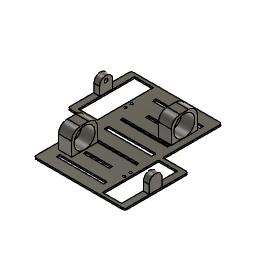
Chassis V4.1 (Autodesk Fusion 360 design; units mm, degrees)
Autodesk Fusion 360 part; units mm, degrees
note: some values were not read from the file. Chosen so that the rebuilt part matches the saved one: which face or edge a step refers to. Set by a fixed rule: which sketch regions a step uses.
sketch "Sketch1" plane through (0, 0, 0) normal (0, 0, 1) x (1, 0, 0)
  line L0 (0, 0) -> (135, 0)
  line L1 (135, 0) -> (135, 150)
  line L2 (135, 150) -> (0, 150)
  line L3 (0, 150) -> (0, 0)
  dimension "d1" = 135
  dimension "d2" = 150
  constraint horizontal L0
  constraint vertical L1
  constraint horizontal L2
  constraint vertical L3
  constraint coincident L0.start L3.end
  measures "d1" distance of L0.start L0.end
  measures "d2" distance of L0.start L2.end
extrude "Extrude1" add sketch "Sketch1" along normal blind 1.75 makes body 1
sketch "Sketch2" plane through (0, 0, 1.75) normal (0, 0, 1) x (-1, 0, 0)
  line L0 (0, -150) -> (0, 0)
  line L1 (0, 0) -> (-135, 0)
  line L2 (-135, 0) -> (-135, -150)
  line L3 (-135, -150) -> (0, -150)
  line L4 (-7.5, -7.5) -> (-127.5, -7.5)
  line L5 (-127.5, -7.5) -> (-127.5, -142.5)
  line L6 (-127.5, -142.5) -> (-7.5, -142.5)
  line L7 (-7.5, -142.5) -> (-7.5, -7.5)
  line L8 (-7.5, -142.5) -> (-29.5, -142.5)
  line L9 (-29.5, -142.5) -> (-29.5, -77.5)
  line L10 (-29.5, -77.5) -> (-7.5, -77.5)
  line L11 (-7.5, -77.5) -> (-7.5, -142.5)
  line L12 (-127.5, -142.5) -> (-127.5, -77.5)
  line L13 (-105.5, -142.5) -> (-127.5, -142.5)
  line L14 (-127.5, -77.5) -> (-105.5, -77.5)
  line L15 (-105.5, -77.5) -> (-105.5, -142.5)
  line L16 (-29.5, -72.5) -> (-29.5, -7.5)
  line L17 (-7.5, -72.5) -> (-29.5, -72.5)
  line L18 (-29.5, -7.5) -> (-7.5, -7.5)
  line L19 (-7.5, -7.5) -> (-7.5, -72.5)
  line L20 (-127.5, -72.5) -> (-127.5, -7.5)
  line L21 (-105.5, -72.5) -> (-127.5, -72.5)
  line L22 (-127.5, -7.5) -> (-105.5, -7.5)
  line L23 (-105.5, -7.5) -> (-105.5, -72.5)
  dimension "d5" = -7.5
  dimension "d6" = 22
  dimension "d7" = 65
  dimension "d10" = -98
  dimension "d11" = 70
  constraint horizontal L8
  constraint vertical L9
  constraint horizontal L10
  constraint vertical L11
  measures "d6" distance of L6.end L8.end
  measures "d7" distance of L6.end L10.end
extrude "Extrude2" cut sketch "Sketch2" against normal up to surface (1.75 mm away) contours L4 L7 L16 L17 L18 L19 | L4 L5 L20 L21 L22 L23 | L6 L7 L8 L9 L10 L11 | L5 L6 L12 L13 L14 L15 bodies 1
sketch "Sketch3" plane through (0, 0, 1.75) normal (0, 0, 1) x (-1, 0, 0)
  line L0 (-127.5, -72.5) -> (-127.5, -7.5)
  line L1 (-127.5, -7.5) -> (-105.5, -7.5)
  line L2 (-105.5, -142.5) -> (-127.5, -142.5)
  line L3 (-127.5, -142.5) -> (-127.5, -77.5)
  line L4 (-127.5, -77.5) -> (-105.5, -77.5)
  line L5 (-7.5, -77.5) -> (-7.5, -142.5)
  line L6 (-7.5, -142.5) -> (-29.5, -142.5)
  line L7 (-29.5, -142.5) -> (-29.5, -77.5)
  line L8 (-29.5, -77.5) -> (-7.5, -77.5)
  line L9 (-7.5, -7.5) -> (-7.5, -72.5)
  line L10 (-29.5, -72.5) -> (-29.5, -7.5)
  line L11 (-29.5, -7.5) -> (-7.5, -7.5)
  line L12 (0, -150) -> (0, 0)
  line L13 (0, 0) -> (-135, 0)
  line L14 (-135, 0) -> (-135, -150)
  line L15 (-135, -150) -> (0, -150)
  line L16 (-29.5, -110) -> (-110.5, -110) construction
  line L17 (-29.5, -40) -> (-110.5, -40) construction
  line L18 (-29.5, -110) -> (-33.25, -110) construction
  line L19 (-30.0705, -117.5) -> (-36.4295, -117.5)
  line L20 (-36.4295, -117.5) -> (-36.4295, -102.5)
  line L21 (-36.4295, -102.5) -> (-30.0705, -102.5)
  line L22 (-30.0705, -102.5) -> (-30.0705, -117.5)
  line L23 (-30.0705, -117.5) -> (-36.4295, -102.5) construction
  line L24 (-36.4295, -117.5) -> (-30.0705, -102.5) construction
  line L25 (-98.5705, -47.5) -> (-104.9295, -47.5)
  line L26 (-98.5705, -32.5) -> (-98.5705, -47.5)
  line L27 (-104.9295, -32.5) -> (-98.5705, -32.5)
  line L28 (-104.9295, -47.5) -> (-104.9295, -32.5)
  line L29 (-110.5, -110) -> (-135, -110) construction
  line L30 (-33.25, -117.5) -> (-33.25, -110) construction
  line L31 (-33.25, -110) -> (-33.25, -102.5) construction
  circle A0 centre (-33.25, -113.75) radius 1.5
  circle A1 centre (-33.25, -106.25) radius 1.5
  line L32 (-101.75, -47.5) -> (-101.75, -40) construction
  line L33 (-101.75, -40) -> (-101.75, -32.5) construction
  circle A2 centre (-101.75, -43.75) radius 1.5
  circle A3 centre (-101.75, -36.25) radius 1.5
  line L34 (-7.5, -110) -> (0, -110) construction
  line L35 (-7.0568, -117.5) -> (-0.4432, -117.5)
  line L36 (-0.4432, -117.5) -> (-0.4432, -102.5)
  line L37 (-0.4432, -102.5) -> (-7.0568, -102.5)
  line L38 (-7.0568, -102.5) -> (-7.0568, -117.5)
  line L39 (-7.0568, -117.5) -> (-0.4432, -102.5) construction
  line L40 (-0.4432, -117.5) -> (-7.0568, -102.5) construction
  line L41 (-134.5568, -47.5) -> (-127.9432, -47.5)
  line L42 (-134.5568, -32.5) -> (-134.5568, -47.5)
  line L43 (-127.9432, -32.5) -> (-134.5568, -32.5)
  line L44 (-127.9432, -47.5) -> (-127.9432, -32.5)
  line L45 (-105.5, -72.5) -> (-127.5, -72.5)
  line L46 (-7.5, -72.5) -> (-29.5, -72.5)
  line L47 (-105.5, -77.5) -> (-105.5, -142.5)
  line L48 (-105.5, -7.5) -> (-105.5, -72.5)
  point P0 (-33.25, -110)
  point P1 (-3.75, -110)
  dimension "d14" = 3.75
  dimension "d15" = 15
  dimension "d18" = -68.5
  dimension "d19" = 70
  dimension "d26" = 3
  dimension "d27" = 3
  dimension "d28" = 3
  dimension "d29" = 3
  dimension "d49" = 15
  dimension "d52" = -127.5
  dimension "d53" = 70
  constraint midpoint L7 L16.start
  constraint midpoint L10 L17.start
  constraint perpendicular L7 L18
  constraint horizontal L19
  constraint perpendicular L19 L20
  constraint parallel L19 L21
  constraint parallel L20 L22
  constraint coincident L23 P0
  constraint coincident L24 P0
  constraint coincident P0 L18.end
  constraint coincident L14 L29.end
  constraint perpendicular L14 L29
  constraint midpoint L19 L30.start
  constraint midpoint L21 L31.end
  constraint midpoint L30 A0.centre
  constraint midpoint L31 A1.centre
  constraint midpoint L25 L32.start
  constraint coincident L17 L32.end
  constraint perpendicular L17 L32
  constraint midpoint L27 L33.end
  constraint midpoint L32 A2.centre
  constraint midpoint L33 A3.centre
  constraint midpoint L5 L34.start
  constraint coincident L12 L34.end
  constraint perpendicular L12 L34
  constraint horizontal L35
  constraint perpendicular L35 L36
  constraint parallel L35 L37
  constraint parallel L36 L38
  constraint coincident L39 P1
  constraint coincident L40 P1
  constraint midpoint L34 P1
  measures "d14" distance of L16.start P0
  measures "d15" distance of L19.end L20.end
  measures "d26" diameter of A0
  measures "d27" diameter of A1
  measures "d28" diameter of A2
  measures "d29" diameter of A3
  measures "d49" distance of L35.end L36.end
extrude "Extrude3" add sketch "Sketch3" along normal blind 17.5 contours L35 L36 L37 L38 | L41 L42 L43 L44 bodies 1
extrude "Extrude4" cut sketch "Sketch3" against normal up to surface (1.75 mm away) contours A0 | A1 | A2 | A3 bodies 1
sketch "Sketch4" plane through (127.5, 0, 0) normal (-1, 0, 0) x (0, -1, 0)
  line L0 (-72.5, 0) -> (-7.5, 0)
  line L1 (-7.5, 0) -> (-7.5, 1.75)
  line L2 (-72.5, 1.75) -> (-7.5, 1.75) construction
  line L3 (-40, 1.75) -> (-40, 13.875) construction
  circle A0 centre (-40, 13.875) radius 2.15
  line L4 (-72.5, 1.75) -> (-72.5, 0)
  line L5 (-7.5, 1.75) -> (-72.5, 1.75)
  dimension "d32" = 12.125
  dimension "d33" = 4.3
  constraint midpoint L2 L3.start
  constraint coincident L3.end A0.centre
  measures "d32" distance of L3.start L3.end
  measures "d33" diameter of A0
sketch "Sketch5" plane through (7.5, 0, 0) normal (1, 0, 0) x (0, 1, 0)
  line L0 (77.5, 0) -> (142.5, 0)
  line L1 (142.5, 0) -> (142.5, 1.75)
  line L2 (77.5, 1.75) -> (77.5, 0)
  line L3 (110, 1.75) -> (110, 13.875) construction
  circle A0 centre (110, 13.875) radius 2.15
  line L4 (142.5, 1.75) -> (77.5, 1.75)
  dimension "d34" = 12.125
  dimension "d35" = 4.3
  constraint coincident L3.end A0.centre
  constraint midpoint L3.start L4
  constraint perpendicular L3 L4
  measures "d34" distance of L3.start L3.end
  measures "d35" diameter of A0
extrude "Extrude5" cut sketch "Sketch5" against normal blind 5 contours A0 bodies 1
extrude "Extrude6" cut sketch "Sketch4" against normal blind 5 contours A0 bodies 1
sketch "Sketch6" plane through (0, 0, 1.75) normal (0, 0, 1) x (-1, 0, 0)
  line L0 (-107.9876, -110) -> (-100.4877, -110.0388) construction
  line L1 (-100.4877, -110.0388) -> (-80.4879, -109.9612) construction
  line L2 (-97.9878, -125) -> (-82.9878, -125)
  line L3 (-82.9878, -125) -> (-82.9878, -95)
  line L4 (-82.9878, -95) -> (-97.9878, -95)
  line L5 (-97.9878, -95) -> (-97.9878, -125)
  line L6 (-97.9878, -125) -> (-82.9878, -95) construction
  line L7 (-82.9878, -125) -> (-97.9878, -95) construction
  line L8 (0, 0) -> (-135, 0)
  line L9 (-69.9889, -150) -> (-67.5, 0) construction
  line L10 (0, -150) -> (0, 0)
  line L11 (-135, 0) -> (-135, -150)
  line L12 (0, -75) -> (-135, -75) construction
  line L13 (-51.9878, -55) -> (-36.9878, -55)
  line L14 (-51.9878, -25) -> (-51.9878, -55)
  line L15 (-36.9878, -25) -> (-51.9878, -25)
  line L16 (-36.9878, -55) -> (-36.9878, -25)
  line L17 (-29.5, -110) -> (-37, -110) construction
  line L18 (-37, -110) -> (-107.9876, -110) construction
  point P0 (-90.4878, -110)
  dimension "d40" = 7.5
  dimension "d41" = 20
  dimension "d42" = 15
  dimension "d43" = 30
  dimension "d46" = 46
  dimension "d47" = 70
  dimension "d48" = 7.5
  constraint horizontal L2
  constraint perpendicular L2 L3
  constraint parallel L2 L4
  constraint parallel L3 L5
  constraint coincident L6 P0
  constraint coincident L7 P0
  constraint midpoint L1 P0
  constraint midpoint L8 L9.end
  constraint midpoint L10 L12.start
  constraint midpoint L11 L12.end
  constraint perpendicular L5 L18
  measures "d40" distance of L0.end L0.start
  measures "d41" distance of L0.end L1.end
  measures "d42" distance of L3.end L4.end
  measures "d43" distance of L2.end L3.end
  measures "d48" distance of L17.start L17.end
extrude "Extrude7" add sketch "Sketch6" along normal blind 26 bodies 1
sketch "Sketch7" plane through (51.9878, 0, 0) normal (1, 0, 0) x (0, 1, 0)
  line L0 (25, 1.75) -> (55, 1.75)
  line L1 (55, 1.75) -> (55, 27.75)
  line L2 (55, 27.75) -> (25, 27.75)
  line L3 (25, 27.75) -> (25, 1.75)
  line L4 (40, 1.75) -> (40, 26) construction
  circle A0 centre (40, 13.875) radius 12.125
  dimension "d56" = 24.25
  dimension "d57" = 24.25
  constraint midpoint L0 L4.start
  constraint perpendicular L0 L4
  constraint midpoint L4 A0.centre
  measures "d56" distance of L4.start L4.end
  measures "d57" diameter of A0
sketch "Sketch8" plane through (82.9878, 0, 0) normal (-1, 0, 0) x (0, -1, 0)
  line L0 (-125, 1.75) -> (-95, 1.75)
  line L1 (-95, 1.75) -> (-95, 27.75)
  line L2 (-95, 27.75) -> (-125, 27.75)
  line L3 (-125, 27.75) -> (-125, 1.75)
  line L4 (-110, 1.75) -> (-110, 26) construction
  circle A0 centre (-110, 13.875) radius 12.125
  dimension "d58" = 24.25
  dimension "d59" = 24.25
  constraint midpoint L0 L4.start
  constraint perpendicular L0 L4
  constraint midpoint L4 A0.centre
  measures "d58" distance of L4.start L4.end
  measures "d59" diameter of A0
extrude "Extrude8" cut sketch "Sketch8" against normal up to surface (15 mm away) contours A0 bodies 1
extrude "Extrude9" cut sketch "Sketch7" against normal blind 15 contours A0 bodies 1
fillet "Fillet1" [suppressed]
fillet "Fillet4" radius 10 4 edges at (90.4878, 95, 27.75) (90.4878, 125, 27.75) (44.4878, 55, 27.75) (44.4878, 25, 27.75) on bodies 1
fillet "Fillet5" radius 7.5 4 edges at (131.25, 47.5, 19.25) (131.25, 32.5, 19.25) (3.75, 102.5, 19.25) (3.75, 117.5, 19.25) on bodies 1
sketch "Sketch9" plane through (0, 0, 0) normal (0, 0, -1) x (1, 0, 0)
  circle A0 centre (33.25, -106.25) radius 1.5
  circle A1 centre (33.25, -113.75) radius 1.5
  line L0 (105.5, -77.5) -> (127.5, -77.5)
  line L1 (127.5, -77.5) -> (127.5, -142.5)
  line L2 (127.5, -142.5) -> (105.5, -142.5)
  line L3 (7.5, -72.5) -> (7.5, -7.5)
  line L4 (7.5, -7.5) -> (29.5, -7.5)
  line L5 (29.5, -7.5) -> (29.5, -72.5)
  line L6 (29.5, -72.5) -> (7.5, -72.5)
  line L7 (105.5, -7.5) -> (127.5, -7.5)
  line L8 (127.5, -7.5) -> (127.5, -72.5)
  line L9 (127.5, -72.5) -> (105.5, -72.5)
  line L10 (7.5, -142.5) -> (7.5, -77.5)
  line L11 (7.5, -77.5) -> (29.5, -77.5)
  line L12 (29.5, -77.5) -> (29.5, -142.5)
  line L13 (29.5, -142.5) -> (7.5, -142.5)
  line L14 (70, 0) -> (70, -150) construction
  line L15 (0, -75) -> (140, -75) construction
  line L16 (0, 0) -> (0, -75) construction
  line L17 (0, 0) -> (0, -75) construction
  line L18 (0, -37.5) -> (140, -37.5) construction
  line L19 (0, -75) -> (0, -145) construction
  line L20 (0, -110) -> (140, -110) construction
  line L21 (85, -35.75) -> (55, -35.75)
  line L22 (55, -35.75) -> (55, -39.25)
  line L23 (55, -39.25) -> (85, -39.25)
  line L24 (85, -39.25) -> (85, -35.75)
  line L25 (85, -35.75) -> (55, -39.25) construction
  line L26 (55, -35.75) -> (85, -39.25) construction
  line L27 (97.5, -72.5) -> (42.5, -72.5)
  line L28 (42.5, -72.5) -> (42.5, -77.5)
  line L29 (42.5, -77.5) -> (97.5, -77.5)
  line L30 (97.5, -77.5) -> (97.5, -72.5)
  line L31 (97.5, -72.5) -> (42.5, -77.5) construction
  line L32 (42.5, -72.5) -> (97.5, -77.5) construction
  line L33 (85, -108.25) -> (55, -108.25)
  line L34 (55, -108.25) -> (55, -111.75)
  line L35 (55, -111.75) -> (85, -111.75)
  line L36 (85, -111.75) -> (85, -108.25)
  line L37 (85, -108.25) -> (55, -111.75) construction
  line L38 (55, -108.25) -> (85, -111.75) construction
  line L39 (0, 0) -> (0, -37.5) construction
  line L40 (0, -37.5) -> (0, -75) construction
  line L41 (0, -75) -> (0, -110) construction
  line L42 (0, -110) -> (0, -151) construction
  line L43 (0, -18.75) -> (140, -18.75) construction
  line L44 (0, -56.25) -> (140, -56.25) construction
  line L45 (0, -92.5) -> (140, -92.5) construction
  line L46 (0, -130.5) -> (140, -130.5) construction
  line L47 (97.5, -54.875) -> (42.5, -54.875)
  line L48 (42.5, -54.875) -> (42.5, -57.625)
  line L49 (42.5, -57.625) -> (97.5, -57.625)
  line L50 (97.5, -57.625) -> (97.5, -54.875)
  line L51 (97.5, -54.875) -> (42.5, -57.625) construction
  line L52 (42.5, -54.875) -> (97.5, -57.625) construction
  line L53 (97.5, -91) -> (42.5, -91)
  line L54 (42.5, -91) -> (42.5, -94)
  line L55 (42.5, -94) -> (97.5, -94)
  line L56 (97.5, -94) -> (97.5, -91)
  line L57 (97.5, -91) -> (42.5, -94) construction
  line L58 (42.5, -91) -> (97.5, -94) construction
  line L59 (97.5, -128.5) -> (42.5, -128.5)
  line L60 (42.5, -128.5) -> (42.5, -132.5)
  line L61 (42.5, -132.5) -> (97.5, -132.5)
  line L62 (97.5, -132.5) -> (97.5, -128.5)
  line L63 (97.5, -128.5) -> (42.5, -132.5) construction
  line L64 (42.5, -128.5) -> (97.5, -132.5) construction
  line L65 (97.5, -16.75) -> (42.5, -16.75)
  line L66 (42.5, -16.75) -> (42.5, -20.75)
  line L67 (42.5, -20.75) -> (97.5, -20.75)
  line L68 (97.5, -20.75) -> (97.5, -16.75)
  line L69 (97.5, -16.75) -> (42.5, -20.75) construction
  line L70 (42.5, -16.75) -> (97.5, -20.75) construction
  line L71 (7.5, -72.5) -> (0, -72.5)
  line L72 (0, -72.5) -> (0, -7.3593)
  line L73 (0, -7.3593) -> (7.5, -7.3593)
  line L74 (7.5, -7.3593) -> (7.5, -72.5)
  line L75 (127.5, -77.5) -> (140, -77.5)
  line L76 (140, -77.5) -> (140, -142.564)
  line L77 (140, -142.564) -> (127.5, -142.564)
  line L78 (127.5, -142.564) -> (127.5, -77.5)
  line L79 (29.5, -7.5) -> (0, -7.5)
  line L80 (0, -7.5) -> (0, 0)
  line L81 (0, 0) -> (29.5, 0)
  line L82 (29.5, 0) -> (29.5, -7.5)
  line L83 (105.5, -142.5) -> (140, -142.5)
  line L84 (140, -142.5) -> (140, -150.5046)
  line L85 (140, -150.5046) -> (105.5, -150.5046)
  line L86 (105.5, -150.5046) -> (105.5, -142.5)
  line L87 (0, -150) -> (135, -150)
  line L88 (135, -150) -> (135, 0)
  line L89 (135, 0) -> (0, 0)
  line L90 (0, 0) -> (0, -150)
  line L91 (105.5, -72.5) -> (105.5, -7.5)
  line L92 (105.5, -142.5) -> (105.5, -77.5)
  circle A2 centre (101.75, -43.75) radius 1.5
  circle A3 centre (101.75, -36.25) radius 1.5
  point P0 (70, -37.5)
  point P1 (70, -75)
  point P2 (70, -110)
  point P3 (70, -56.25)
  point P4 (70, -92.5)
  point P5 (70, -130.5)
  point P6 (70, -18.75)
  dimension "d74" = 30
  dimension "d75" = 3.5
  dimension "d76" = 55
  dimension "d77" = 5
  dimension "d78" = 30
  dimension "d79" = 3.5
  dimension "d82" = 55
  dimension "d83" = 2.75
  dimension "d84" = 55
  dimension "d85" = 3
  dimension "d86" = 55
  dimension "d87" = 4
  dimension "d88" = 55
  dimension "d89" = 4
  constraint coincident L16.start L17.start
  constraint midpoint L17 L18.start
  constraint midpoint L19 L20.start
  constraint horizontal L21
  constraint perpendicular L21 L22
  constraint parallel L21 L23
  constraint parallel L22 L24
  constraint coincident L25 P0
  constraint coincident L26 P0
  constraint midpoint L18 P0
  constraint horizontal L27
  constraint perpendicular L27 L28
  constraint parallel L27 L29
  constraint parallel L28 L30
  constraint coincident L31 P1
  constraint coincident L32 P1
  constraint midpoint L14 P1
  constraint horizontal L33
  constraint perpendicular L33 L34
  constraint parallel L33 L35
  constraint parallel L34 L36
  constraint coincident L37 P2
  constraint coincident L38 P2
  constraint midpoint L20 P2
  constraint midpoint L39 L43.start
  constraint midpoint L40 L44.start
  constraint midpoint L41 L45.start
  constraint midpoint L42 L46.start
  constraint horizontal L47
  constraint perpendicular L47 L48
  constraint parallel L47 L49
  constraint parallel L48 L50
  constraint coincident L51 P3
  constraint coincident L52 P3
  constraint midpoint L44 P3
  constraint horizontal L53
  constraint perpendicular L53 L54
  constraint parallel L53 L55
  constraint parallel L54 L56
  constraint coincident L57 P4
  constraint coincident L58 P4
  constraint midpoint L45 P4
  constraint horizontal L59
  constraint perpendicular L59 L60
  constraint parallel L59 L61
  constraint parallel L60 L62
  constraint coincident L63 P5
  constraint coincident L64 P5
  constraint midpoint L46 P5
  constraint horizontal L65
  constraint perpendicular L65 L66
  constraint parallel L65 L67
  constraint parallel L66 L68
  constraint coincident L69 P6
  constraint coincident L70 P6
  constraint midpoint L43 P6
  constraint horizontal L71
  constraint vertical L72
  constraint horizontal L73
  constraint vertical L74
  constraint coincident L39 L72.end
  constraint coincident L3.start L6.end
  constraint horizontal L75
  constraint vertical L76
  constraint horizontal L77
  constraint vertical L78
  constraint coincident L0.end L1.start
  constraint horizontal L79
  constraint vertical L80
  constraint horizontal L81
  constraint vertical L82
  constraint coincident L4.end L5.start
  constraint horizontal L83
  constraint vertical L84
  constraint horizontal L85
  constraint vertical L86
  constraint coincident L2.end L83.start
  measures "d74" distance of L22.end L23.end
  measures "d75" distance of L21.end L22.end
  measures "d76" distance of L28.end L29.end
  measures "d77" distance of L27.end L28.end
  measures "d78" distance of L34.end L35.end
  measures "d79" distance of L33.end L34.end
  measures "d82" distance of L48.end L49.end
  measures "d83" distance of L47.end L48.end
  measures "d84" distance of L54.end L55.end
  measures "d85" distance of L53.end L54.end
  measures "d86" distance of L60.end L61.end
  measures "d87" distance of L59.end L60.end
  measures "d88" distance of L66.end L67.end
  measures "d89" distance of L65.end L66.end
extrude "Extrude10" cut sketch "Sketch9" against normal up to surface (1.75 mm away) contours L21 L22 L23 L24 | L27 L28 L29 L30 | L33 L34 L35 L36 | L47 L48 L49 L50 | L53 L54 L55 L56 | L59 L60 L61 L62 | L65 L66 L67 L68 bodies 1
extrude "Extrude11" cut sketch "Sketch9" against normal up to surface (1.75 mm away) contours L1 L75 L78 L83 L88 | L2 L77 L78 L83 L86 L87 L88 | L77 L78 L83 L88 | L77 L84 L85 L86 L87 L88 | L4 L73 L74 L79 L80 L81 L82 L89 L90 | L3 L71 L72 L74 L79 L90 | L72 L73 L74 L79 L80 L90 bodies 1
fillet "Fillet6" [suppressed]
sketch "Sketch10" plane through (0, 0, 0) normal (0, 0, -1) x (1, 0, 0)
  line L0 (0, -72.5) -> (0, -150)
  line L1 (0, -150) -> (105.5, -150)
  line L2 (105.5, -150) -> (105.5, -77.5)
  line L3 (105.5, -77.5) -> (135, -77.5)
  line L4 (135, -77.5) -> (135, 0)
  line L5 (135, 0) -> (29.5, 0)
  line L6 (29.5, 0) -> (29.5, -72.5)
  line L7 (29.5, -72.5) -> (0, -72.5)
  line L8 (7.5, -142.5) -> (7.5, -77.5)
  line L9 (7.5, -77.5) -> (29.5, -77.5)
  line L10 (29.5, -77.5) -> (29.5, -142.5)
  line L11 (29.5, -142.5) -> (7.5, -142.5)
  line L12 (105.5, -7.5) -> (127.5, -7.5)
  line L13 (127.5, -7.5) -> (127.5, -72.5)
  line L14 (127.5, -72.5) -> (105.5, -72.5)
  circle A0 centre (33.25, -113.75) radius 1.5
  circle A1 centre (33.25, -106.25) radius 1.5
  line L15 (97.5, -132.5) -> (42.5, -132.5)
  line L16 (42.5, -132.5) -> (42.5, -128.5)
  line L17 (42.5, -128.5) -> (97.5, -128.5)
  line L18 (97.5, -128.5) -> (97.5, -132.5)
  line L19 (85, -111.75) -> (55, -111.75)
  line L20 (55, -111.75) -> (55, -108.25)
  line L21 (55, -108.25) -> (85, -108.25)
  line L22 (85, -108.25) -> (85, -111.75)
  line L23 (97.5, -77.5) -> (42.5, -77.5)
  line L24 (42.5, -77.5) -> (42.5, -72.5)
  line L25 (42.5, -72.5) -> (97.5, -72.5)
  line L26 (97.5, -72.5) -> (97.5, -77.5)
  line L27 (97.5, -94) -> (42.5, -94)
  line L28 (42.5, -94) -> (42.5, -91)
  line L29 (42.5, -91) -> (97.5, -91)
  line L30 (97.5, -91) -> (97.5, -94)
  line L31 (97.5, -20.75) -> (42.5, -20.75)
  line L32 (42.5, -20.75) -> (42.5, -16.75)
  line L33 (42.5, -16.75) -> (97.5, -16.75)
  line L34 (97.5, -16.75) -> (97.5, -20.75)
  line L35 (85, -39.25) -> (55, -39.25)
  line L36 (55, -39.25) -> (55, -35.75)
  line L37 (55, -35.75) -> (85, -35.75)
  line L38 (85, -35.75) -> (85, -39.25)
  line L39 (97.5, -57.625) -> (42.5, -57.625)
  line L40 (42.5, -57.625) -> (42.5, -54.875)
  line L41 (42.5, -54.875) -> (97.5, -54.875)
  line L42 (97.5, -54.875) -> (97.5, -57.625)
  line L43 (105.5, -7.5) -> (105.5, 0) construction
  line L44 (29.5, -142.5) -> (29.5, -150) construction
  line L45 (29.5, -150) -> (31.5, -150) construction
  line L46 (31.5, -150) -> (36.5, -150)
  line L47 (36.5, -150) -> (36.5, 0)
  line L48 (36.5, 0) -> (31.5, 0)
  line L49 (31.5, 0) -> (31.5, -150)
  line L50 (105.5, 0) -> (103.5, 0) construction
  line L51 (103.5, 0) -> (98.5, 0)
  line L52 (98.5, 0) -> (98.5, -150)
  line L53 (98.5, -150) -> (103.5, -150)
  line L54 (103.5, -150) -> (103.5, 0)
  circle A2 centre (33.25, -113.75) radius 1.75
  circle A3 centre (33.25, -106.25) radius 1.75
  circle A4 centre (106.75, -36.25) radius 1.75
  circle A5 centre (101.75, -43.75) radius 1.75
  line L55 (33.25, -113.75) -> (33.25, -116.75)
  line L56 (33.25, -106.25) -> (33.25, -103.25)
  line L57 (36.5, -103.25) -> (31.5, -103.25)
  line L58 (36.5, -116.75) -> (31.5, -116.75)
  line L59 (106.75, -36.25) -> (106.75, -33.25)
  line L60 (101.75, -43.75) -> (101.75, -46.75)
  line L61 (98.5, -46.75) -> (103.5, -46.75)
  line L62 (98.5, -33.25) -> (103.5, -33.25)
  line L63 (105.5, -72.5) -> (105.5, -7.5)
  circle A6 centre (101.75, -43.75) radius 1.5
  circle A7 centre (101.75, -36.25) radius 1.5
  dimension "d94" = 2
  dimension "d95" = 5
  dimension "d96" = 2
  dimension "d97" = 5
  dimension "d98" = 3.5
  dimension "d99" = 3.5
  dimension "d100" = 3.5
  dimension "d101" = 3.5
  dimension "d108" = 3
  dimension "d109" = 3
  dimension "d110" = 3
  dimension "d111" = 3
  constraint coincident L12.start L43.start
  constraint coincident L5 L43.end
  constraint perpendicular L5 L43
  constraint coincident L10.end L11.start
  constraint coincident L1 L44.end
  constraint perpendicular L1 L44
  constraint perpendicular L44 L45
  constraint horizontal L46
  constraint vertical L47
  constraint horizontal L48
  constraint vertical L49
  constraint perpendicular L43 L50
  constraint horizontal L51
  constraint vertical L52
  constraint horizontal L53
  constraint vertical L54
  constraint concentric A0 A2
  constraint concentric A1 A3
  constraint concentric A5 A6
  constraint coincident A0.centre A2.centre
  constraint parallel L47 L55
  constraint coincident A1.centre A3.centre
  constraint vertical L56
  constraint coincident L47 L57.start
  constraint coincident L49 L57.end
  constraint perpendicular L49 L57
  constraint coincident L47 L58.start
  constraint coincident L49 L58.end
  constraint perpendicular L49 L58
  constraint vertical L59
  constraint coincident A5.centre L60.start
  constraint vertical L60
  constraint coincident L52 L61.start
  constraint coincident L54 L61.end
  constraint perpendicular L54 L61
  constraint coincident L52 L62.start
  constraint coincident L54 L62.end
  constraint perpendicular L54 L62
  measures "d94" distance of L44.end L45.end
  measures "d95" distance of L45.end L46.end
  measures "d96" distance of L43.end L50.end
  measures "d97" distance of L50.end L51.end
  measures "d98" diameter of A2
  measures "d99" diameter of A3
  measures "d100" diameter of A4
  measures "d101" diameter of A5
  measures "d108" distance of A0.centre L55.end
  measures "d109" distance of A1.centre L56.end
  measures "d110" distance of A4.centre L59.end
  measures "d111" distance of A5.centre L60.end
extrude "Extrude12" add sketch "Sketch10" along normal blind 1 separate body contours L1 L46 L47 L49 L58 | L5 L47 L48 L49 L57 | L1 L52 L53 L54 L61 | L5 L51 L52 L54 L62 makes body 2 at (33.1667, 34.4167, 0) makes body 3 at (34.8333, 127.8333, 0) makes body 4 at (100.1667, 11.0833, 0) makes body 5 at (100.1667, 81.1667, 0)
sketch "Sketch11" plane through (0, 0, -1) normal (0, 0, -1) x (1, 0, 0)
  line L0 (103.2773, 0) -> (102.2773, 0)
  line L1 (102.2773, 0) -> (102.2773, -150)
  line L2 (102.2773, -150) -> (103.2773, -150)
  line L3 (103.2773, -150) -> (103.2773, 0)
  line L4 (120.5, 0) -> (103.5, -46.75)
  line L5 (103.5, -33.25) -> (98.5, -33.25)
  line L6 (103.5, -46.75) -> (102.2773, -46.75)
  line L7 (103.5, -33.25) -> (102.2773, -33.25)
  line L8 (98.5, 0) -> (98.5, -33.25)
  line L9 (98.5, -33.25) -> (103.5, -33.25)
  line L10 (103.5, -33.25) -> (103.5, 0)
  line L11 (103.5, 0) -> (98.5, 0)
  line L12 (98.5, -150) -> (103.5, -150)
  line L13 (103.5, -150) -> (103.5, -46.75)
  line L14 (103.5, -46.75) -> (98.5, -46.75)
  line L15 (98.5, -46.75) -> (98.5, -150)
  point P0 (103.5, -33.25)
  point P1 (98.5, -33.25)
  dimension "d104" = 1
  constraint horizontal L0
  constraint vertical L1
  constraint horizontal L2
  constraint vertical L3
  constraint coincident P0 L5.start
  constraint coincident P1 L5.end
  constraint coincident L1 L6.end
  constraint coincident L1 L7.end
  constraint coincident L5 L7.end
  measures "d104" distance of L0.start L0.end
sketch "Sketch12" plane through (0, 0, -1) normal (0, 0, -1) x (1, 0, 0)
  line L0 (31.5, -150) -> (32.5, -150)
  line L1 (32.5, -150) -> (32.5, 0)
  line L2 (32.5, 0) -> (31.5, 0)
  line L3 (31.5, 0) -> (31.5, -150)
  line L4 (31.5, -116.75) -> (36.5, -116.75)
  line L5 (31.5, -103.25) -> (36.5, -103.25)
  line L6 (36.5, -116.75) -> (31.5, -116.75)
  line L7 (31.5, -116.75) -> (31.5, -150)
  line L8 (31.5, -150) -> (36.5, -150)
  line L9 (36.5, -103.25) -> (36.5, 0)
  line L10 (36.5, 0) -> (31.5, 0)
  line L11 (31.5, 0) -> (31.5, -103.25)
  line L12 (31.5, -103.25) -> (36.5, -103.25)
  line L13 (36.5, -150) -> (36.5, -116.75)
  point P0 (31.5, -116.75)
  point P1 (36.5, -116.75)
  dimension "d105" = 1
  constraint horizontal L0
  constraint vertical L1
  constraint horizontal L2
  constraint vertical L3
  constraint coincident P0 L4.start
  constraint coincident P1 L4.end
  measures "d105" distance of L0.start L0.end
extrude "Extrude14" add sketch "Sketch12" sketch "Sketch11" along normal blind 15 contours L0 L1 L3 L4 L6 L7 L8 | L1 L2 L3 L5 L10 L11 L12 of sketch 2 contours L0 L1 L3 L5 L7 L9 L11 | L1 L2 L3 L6 L12 L14 bodies 3 4 2 makes body 6
sketch "Sketch13" plane through (0, 0, 1.75) normal (0, 0, 1) x (-1, 0, 0)
  line L0 (-97.5, -54.875) -> (-51.9878, -54.875)
  line L1 (-51.9878, -54.875) -> (-51.9878, -40)
  line L2 (-51.9878, -40) -> (-51.9878, -25)
  line L3 (-51.9878, -25) -> (-36.9878, -25)
  line L4 (-36.9878, -25) -> (-36.9878, -40)
  line L5 (-36.9878, -40) -> (-36.9878, -55)
  line L6 (-36.9878, -55) -> (-42.5, -55)
  line L7 (-42.5, -55) -> (-42.5, -57.625)
  line L8 (-42.5, -57.625) -> (-97.5, -57.625)
  line L9 (-97.5, -57.625) -> (-97.5, -54.875)
  line L10 (-55, -39.25) -> (-85, -39.25)
  line L11 (-85, -39.25) -> (-85, -35.75)
  line L12 (-85, -35.75) -> (-55, -35.75)
  line L13 (-55, -35.75) -> (-55, -39.25)
  line L14 (-42.5, -20.75) -> (-97.5, -20.75)
  line L15 (-97.5, -20.75) -> (-97.5, -16.75)
  line L16 (-97.5, -16.75) -> (-42.5, -16.75)
  line L17 (-42.5, -16.75) -> (-42.5, -20.75)
  line L18 (-42.5, -94) -> (-97.5, -94)
  line L19 (-97.5, -94) -> (-97.5, -91)
  line L20 (-97.5, -91) -> (-42.5, -91)
  line L21 (-42.5, -91) -> (-42.5, -94)
  line L22 (-42.5, -77.5) -> (-97.5, -77.5)
  line L23 (-97.5, -77.5) -> (-97.5, -72.5)
  line L24 (-97.5, -72.5) -> (-42.5, -72.5)
  line L25 (-42.5, -72.5) -> (-42.5, -77.5)
  line L26 (-55, -111.75) -> (-82.9878, -111.75)
  line L27 (-82.9878, -108.25) -> (-55, -108.25)
  line L28 (-55, -108.25) -> (-55, -111.75)
  line L29 (-42.5, -132.5) -> (-97.5, -132.5)
  line L30 (-97.5, -132.5) -> (-97.5, -128.5)
  line L31 (-97.5, -128.5) -> (-42.5, -128.5)
  line L32 (-42.5, -128.5) -> (-42.5, -132.5)
  line L33 (-97.9878, -95) -> (-82.9878, -95)
  line L34 (-82.9878, -111.75) -> (-82.9878, -125)
  line L35 (-82.9878, -125) -> (-97.9878, -125)
  line L36 (-97.9878, -125) -> (-97.9878, -110)
  line L37 (-97.9878, -110) -> (-97.9878, -95)
  circle A0 centre (-33.25, -106.25) radius 1.5
  circle A1 centre (-33.25, -113.75) radius 1.5
  line L38 (-7.0568, -102.5) -> (-0.4432, -102.5)
  line L39 (-0.4432, -102.5) -> (-0.4432, -117.5)
  line L40 (-0.4432, -117.5) -> (-7.0568, -117.5)
  line L41 (-7.0568, -117.5) -> (-7.0568, -102.5)
  line L42 (-127.9432, -47.5) -> (-134.5568, -47.5)
  line L43 (-134.5568, -32.5) -> (-127.9432, -32.5)
  line L44 (-127.9432, -32.5) -> (-127.9432, -47.5)
  line L45 (-105.5, -72.5) -> (-127.5, -72.5)
  line L46 (-127.5, -72.5) -> (-127.5, -7.5)
  line L47 (-127.5, -7.5) -> (-105.5, -7.5)
  line L48 (-7.5, -77.5) -> (-7.5, -142.5)
  line L49 (-7.5, -142.5) -> (-29.5, -142.5)
  line L50 (-29.5, -142.5) -> (-29.5, -77.5)
  line L51 (-29.5, -77.5) -> (-7.5, -77.5)
  line L52 (0, -72.5) -> (-29.5, -72.5)
  line L53 (-29.5, -72.5) -> (-29.5, 0)
  line L54 (-29.5, 0) -> (-135, 0)
  line L55 (-135, 0) -> (-135, -77.5)
  line L56 (-135, -77.5) -> (-105.5, -77.5)
  line L57 (-105.5, -77.5) -> (-105.5, -150)
  line L58 (-105.5, -150) -> (0, -150)
  line L59 (0, -150) -> (0, -72.5)
  line L60 (-105.5, -7.5) -> (-105.5, -72.5)
  line L61 (-134.5568, -47.5) -> (-134.5568, -32.5)
  circle A2 centre (-101.75, -36.25) radius 1.5
  circle A3 centre (-101.75, -43.75) radius 1.5
  line L62 (-82.9878, -95) -> (-82.9878, -108.25)
sketch "Sketch14" plane through (0, 0, 1.75) normal (0, 0, 1) x (-1, 0, 0)
  line L0 (-29.5, 0) -> (-29.5, -3.75) construction
  line L1 (-105.5, -150) -> (-105.5, -146.25) construction
  line L2 (0, -150) -> (0, -72.5)
  line L3 (-105.5, -146.25) -> (0, -146.25)
  line L4 (-135, 0) -> (-135, -77.5)
  line L5 (-29.5, -3.75) -> (-135, -3.75)
  line L6 (0, -146.25) -> (-105.5, -146.25)
  line L7 (-105.5, -146.25) -> (-105.5, -150)
  line L8 (-105.5, -150) -> (0, -150)
  line L9 (0, -150) -> (0, -146.25)
  line L10 (-29.5, 0) -> (-135, 0)
  line L11 (-135, 0) -> (-135, -3.75)
  line L12 (-135, -3.75) -> (-29.5, -3.75)
  line L13 (-29.5, -3.75) -> (-29.5, 0)
  point P0 (-29.5, 0)
  point P1 (-105.5, -150)
  dimension "d114" = 3.75
  dimension "d115" = 3.75
  constraint coincident P0 L0.start
  constraint coincident P1 L1.start
  constraint coincident L2 L3.end
  constraint perpendicular L1 L3
  constraint coincident L4 L5.end
  constraint perpendicular L0 L5
  constraint horizontal L6
  constraint vertical L7
  constraint horizontal L8
  constraint vertical L9
  constraint horizontal L10
  constraint vertical L11
  constraint horizontal L12
  constraint vertical L13
  measures "d114" distance of P0 L0.end
  measures "d115" distance of P1 L1.end
extrude "Extrude15" cut sketch "Sketch14" against normal up to surface (1.75 mm away) bodies 1
fillet "Fillet7" radius 2.5 6 edges at (29.5, 3.75, 0.875) (135, 3.75, 0.875) (135, 77.5, 0.875) (105.5, 146.25, 0.875) (0, 146.25, 0.875) (0, 72.5, 0.875) on bodies 1
hidden bodies 3 4 2 5 6
